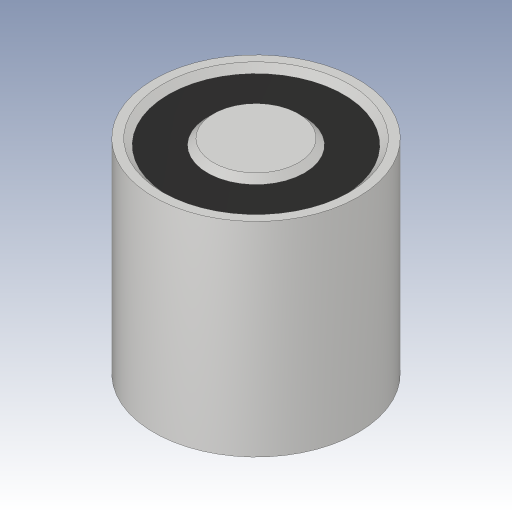
# Autodesk Inventor part: Nummer?
Saved by Autodesk Inventor 2023.3 (Build 273359000, 359)
## iProperties
Company: HTBLA Kaindorf
RuleStatus: InUse
Created: 2024-01-29
Part Number: Nummer?
Project: Fiberprinter-Hotend
Material: Aluminium
Description: Bauteilname?
Document SubType Name: Modeling
Designer: Konstrukteur?
Mass: 3.51807 g
Surface Area: 7.36085 cm^2
Volume: 1.30299 cm^3
Density: 2.7 g/cm^3
Appearance: Satin
AfterDocNew0: iProperties-Editor_aufrufen
Author: nicob
Keywords: Schuljahr?
Autodesk Inventor part; units mm, degrees
ref_plane "YZ Plane" through (0, 0, 0) normal (1, 0, 0) x (0, 1, 0)
ref_plane "XZ Plane" through (0, 0, 0) normal (0, 1, 0) x (-1, 0, 0)
ref_plane "XY Plane" through (0, 0, 0) normal (0, 0, 1) x (1, 0, 0)
sketch "Skizze3" plane through (0, 0, 0) normal (1, 0, 0) x (0, 1, 0)
  line L0 (0, 0) -> (0, 20.035)
  line L1 (0, 0) -> (6, 0)
  line L2 (6, 0) -> (6, 12)
  line L3 (6, 12) -> (5.5, 12)
  line L4 (5.5, 12) -> (5.5, 11.65)
  line L5 (5.5, 11.65) -> (2.5, 11.65)
  line L6 (2.5, 11.65) -> (2.5, 12)
  line L7 (2.5, 12) -> (0, 12)
  point P0 (2.5, 11.825)
  dimension "d4" = 6
  dimension "d5" = 12
  dimension "d6" = 5
  dimension "d7" = 3
  dimension "d8" = 0.35
  constraints: 16 end point, 5 perpendicular, 3 point on line, 1 horizontal, 1 midpoint, 1 vertical
  measures "d4" distance of L0.start L1.end
  measures "d5" distance of L1.end L2.end
  measures "d6" diameter of L6 L0
  measures "d7" distance from line of point (2.5, 11.825) L4
  measures "d8" distance between parallel lines of L3 L5
revolve "Umdrehung1" add sketch "Skizze3" angle 360 about axis through (0, 0, 0) along (0, 0, 1)
chamfer "Fase2" distance 0.35 angle 45 2 edges at (0, -5.5, 11.65) (0, -2.5, 11.65)
sketch "Skizze4" plane through (0, 0, 0) normal (0, 0, -1) x (-1, 0, 0)
  circle A0 centre (0, 0) radius 2.5 projected
  constraints: 1 coincident
hole "Bohrung1" at (0, 0, 0) direction (0, 0, 1) diameter 2.459 depth 6.5 start extended yes thread size "M3x0.5" class "6H" standard "ISO Metric profile"
